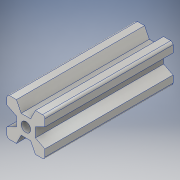
# Autodesk Inventor part: Mock 8020 3.375in
Saved by Autodesk Inventor 2016 (Build 200138000, 138)
## iProperties
Created: 2016-12-12
Part Number: Mock 8020 3.375in
Material: Aluminum 6061
Document SubType Name: Modeling
Designer: Kyle
Density: 2.7 g/cm^3
Appearance: Aluminum - Flat
Author: Kyle
Autodesk Inventor part; units mm, degrees
ref_plane "YZ Plane" through (0, 0, 0) normal (1, 0, 0) x (0, 1, 0)
ref_plane "XZ Plane" through (0, 0, 0) normal (0, 1, 0) x (-1, 0, 0)
ref_plane "XY Plane" through (0, 0, 0) normal (0, 0, 1) x (1, 0, 0)
sketch "Sketch1" plane through (0, 0, 0) normal (0, 0, 1) x (1, 0, 0)
  line L0 (0, 0) -> (25.4, 0)
  line L1 (25.4, 0) -> (25.4, 25.4)
  line L2 (25.4, 25.4) -> (0, 25.4)
  line L3 (0, 25.4) -> (0, 0)
  circle A0 centre (12.7, 12.7) radius 3.175
  dimension "d0" = 25.4
  dimension "d1" = 25.4
  dimension "d2" = 6.35
  dimension "d7" = 12.7
  dimension "d8" = 12.7
  constraints: 8 end point, 2 parallel, 1 centre point, 1 horizontal, 1 perpendicular
  measures "d0" distance of L2.end L1.end
  measures "d1" distance of L1.end L0.end
  measures "d2" diameter of A0
  measures "d7" distance from line of L2 A0.centre
  measures "d8" distance from line of L1 A0.centre
extrude "Extrusion1" add sketch "Sketch1" along normal blind 609.6
sketch "Sketch2" plane through (0, 0, 609.6) normal (0, 0, 1) x (1, 0, 0)
  line L0 (25.4, 25.4) -> (0, 25.4) projected
  line L1 (0, 25.4) -> (0, 0) projected
  circle A0 centre (12.7, 12.7) radius 3.175 projected
  line L2 (0, 0) -> (25.4, 0) projected
  line L3 (25.4, 0) -> (25.4, 25.4) projected
  line L4 (25.4, 25.4) -> (0, 25.4) projected
  line L5 (0, 25.4) -> (0, 0) projected
  line L6 (12.7, 19.05) -> (9.525, 19.05)
  line L7 (9.525, 19.05) -> (15.875, 19.05)
  line L8 (15.875, 19.05) -> (19.05, 25.4)
  line L9 (9.525, 19.05) -> (6.35, 25.4)
  dimension "d13" = 6.35
  dimension "d14" = 6.35
  dimension "d15" = 3.175
  dimension "d16" = 6.35
  constraints: 8 end point, 2 point on line
  measures "d13" distance of L0.start L8.end
  measures "d14" distance of L0.end L9.end
  measures "d15" distance of L6.start L6.end
  measures "d16" distance of L6.end L7.end
fillet "Fillet1" radius 1.5875 4 edges at (25.4, 25.4, 304.8) (0, 25.4, 304.8) (25.4, 0, 304.8) (0, 0, 304.8)
extrude "Extrusion2" cut sketch "Sketch2" against normal blind 609.6 contours L8 L7 L6 L9 L0
pattern_circular "Circular Pattern1" count 4 over 360 about axis through (12.7, 12.7, 0) along (0, 0, 1) of "Extrusion2"
sketch "Sketch3" plane through (0, 0, 609.6) normal (0, 0, 1) x (1, 0, 0)
  line L0 (19.05, 15.875) -> (25.4, 19.05) projected
  line L1 (25.4, 19.05) -> (25.4, 23.8125) projected
  arc A0 (25.4, 23.8125) -> (23.8125, 25.4) centre (23.8125, 23.8125) ccw projected
  line L2 (23.8125, 25.4) -> (19.05, 25.4) projected
  line L3 (19.05, 25.4) -> (15.875, 19.05) projected
  line L4 (15.875, 19.05) -> (9.525, 19.05) projected
  line L5 (9.525, 19.05) -> (6.35, 25.4) projected
  line L6 (6.35, 25.4) -> (1.5875, 25.4) projected
  arc A1 (1.5875, 25.4) -> (0, 23.8125) centre (1.5875, 23.8125) ccw projected
  line L7 (0, 23.8125) -> (0, 19.05) projected
  line L8 (0, 19.05) -> (6.35, 15.875) projected
  line L9 (6.35, 15.875) -> (6.35, 9.525) projected
  line L10 (6.35, 9.525) -> (0, 6.35) projected
  line L11 (0, 6.35) -> (0, 1.5875) projected
  arc A2 (0, 1.5875) -> (1.5875, 0) centre (1.5875, 1.5875) ccw projected
  line L12 (1.5875, 0) -> (6.35, 0) projected
  line L13 (6.35, 0) -> (9.525, 6.35) projected
  line L14 (9.525, 6.35) -> (15.875, 6.35) projected
  line L15 (15.875, 6.35) -> (19.05, 0) projected
  line L16 (19.05, 0) -> (23.8125, 0) projected
  arc A3 (23.8125, 0) -> (25.4, 1.5875) centre (23.8125, 1.5875) ccw projected
  line L17 (25.4, 1.5875) -> (25.4, 6.35) projected
  line L18 (25.4, 6.35) -> (19.05, 9.525) projected
  line L19 (19.05, 9.525) -> (19.05, 15.875) projected
  circle A4 centre (12.7, 12.7) radius 3.175 projected
  point P0 (0, 0)
extrude "Extrusion3" cut sketch "Sketch3" against normal blind 517.525
sketch "Sketch4" plane through (0, 0, 92.075) normal (0, 0, 1) x (1, 0, 0)
  circle A0 centre (12.7, 12.7) radius 3.175 projected
  line L0 (25.4, 19.05) -> (19.05, 15.875) projected
  line L1 (25.4, 23.8125) -> (25.4, 19.05) projected
  arc A1 (25.4, 23.8125) -> (23.8125, 25.4) centre (23.8125, 23.8125) ccw projected
  line L2 (19.05, 25.4) -> (23.8125, 25.4) projected
  line L3 (15.875, 19.05) -> (19.05, 25.4) projected
  line L4 (9.525, 19.05) -> (15.875, 19.05) projected
  line L5 (6.35, 25.4) -> (9.525, 19.05) projected
  line L6 (1.5875, 25.4) -> (6.35, 25.4) projected
  arc A2 (1.5875, 25.4) -> (0, 23.8125) centre (1.5875, 23.8125) ccw projected
  line L7 (0, 19.05) -> (0, 23.8125) projected
  line L8 (6.35, 15.875) -> (0, 19.05) projected
  line L9 (6.35, 9.525) -> (6.35, 15.875) projected
  line L10 (0, 6.35) -> (6.35, 9.525) projected
  line L11 (0, 1.5875) -> (0, 6.35) projected
  arc A3 (0, 1.5875) -> (1.5875, 0) centre (1.5875, 1.5875) ccw projected
  line L12 (6.35, 0) -> (1.5875, 0) projected
  line L13 (9.525, 6.35) -> (6.35, 0) projected
  line L14 (15.875, 6.35) -> (9.525, 6.35) projected
  line L15 (19.05, 0) -> (15.875, 6.35) projected
  line L16 (23.8125, 0) -> (19.05, 0) projected
  arc A4 (23.8125, 0) -> (25.4, 1.5875) centre (23.8125, 1.5875) ccw projected
  line L17 (25.4, 6.35) -> (25.4, 1.5875) projected
  line L18 (19.05, 9.525) -> (25.4, 6.35) projected
  line L19 (19.05, 15.875) -> (19.05, 9.525) projected
  point P0 (0, 0)
extrude "Extrusion4" cut sketch "Sketch4" against normal blind 6.35
body "Solid1"
